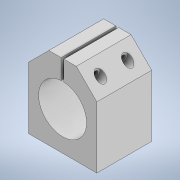
# Autodesk Inventor part: Motor_ParallelMecha_Fixation_Holder
Saved by Autodesk Inventor 2022 (Build 260153000, 153)
## iProperties
Created: 2022-07-26
Part Number: Motor_ParallelMecha_Fixation_Holder
Material: Generisch
Document SubType Name: Modeling
Designer: alexw
Density: 1 g/cm^3
Appearance: Vorgabe
Mass: 35.2121 g
Surface Area: 107.982 cm^2
Volume: 35.2121 cm^3
Hole_Dist2Center: 10,000 mm
Author: alexw
Autodesk Inventor part; units mm, degrees
note: some values were not read from the file. Chosen so that the rebuilt part matches the saved one: direction of "Bohrung2".
sketch "Skizze1" plane through (0, 0, 0) normal (0, 0, 1) x (1, 0, 0)
  line L0 (0, 0) -> (50, 0)
  line L1 (50, 0) -> (50, 45)
  line L2 (35, 60) -> (15, 60)
  line L3 (0, 45) -> (0, 0)
  circle A0 centre (25, 28) radius 17.5
  line L4 (25, 28) -> (25, 0) construction
  line L5 (0, 45) -> (15, 60)
  line L6 (35, 60) -> (50, 45)
  line L7 (24, 60) -> (26, 60)
  line L8 (26, 60) -> (26, 28)
  line L9 (26, 28) -> (24, 28)
  line L10 (24, 28) -> (24, 60)
  point P0 (50, 60)
  point P1 (0, 60)
  point P2 (25, 60)
  dimension "d0" = 50
  dimension "d1" = 35
  dimension "d2" = 60
  dimension "d3" = 15
  dimension "d4" = 15
  dimension "d5" = 15
  dimension "d6" = 15
  dimension "d7" = 28
  dimension "d10" = 2
  constraints: 22 end point, 4 midpoint, 4 parallel, 4 point on line, 2 horizontal, 2 perpendicular, 1 centre point, 1 vertical
  measures "d0" distance between parallel lines of L1 L3
  measures "d1" diameter of A0
  measures "d2" distance between parallel lines of L2 L0
  measures "d3" distance of L3.start point (0, 60)
  measures "d4" distance of L2.end point (0, 60)
  measures "d5" distance of L2.start point (50, 60)
  measures "d6" distance of L1.end point (50, 60)
  measures "d7" distance of L4.start L4.end
  measures "d10" distance between parallel lines of L8 L10
extrude "Extrusion1" add sketch "Skizze1" along normal blind 40 contours L3 L5 L2 L10 A0 L8 L6 L1 L0 | L2 L8 A0 L10
extrude "Extrusion2" cut sketch "Skizze1" along normal up to surface (40 mm away) contours L2 L8 A0 L10 | A0 L8 L9 L10 picked at (24.8888, 33.8323)
sketch "Skizze2" plane through (0, 0, 0) normal (0, -1, 0) x (1, 0, 0)
  line L0 (0, 0) -> (0, 40) construction
  line L1 (50, 0) -> (50, 40) construction
  line L2 (0, 40) -> (50, 40) construction
  line L3 (0, 0) -> (0, 40) construction
  line L4 (25, 20) -> (25, 40) construction
  line L5 (7.5, 40) -> (42.5, 40) construction
  line L6 (11, 20) -> (39, 20) construction
  point P0 (26, 40)
  point P1 (24, 40)
  point P2 (0, 20)
  dimension "d13" = 28
  constraints: 4 end point, 3 midpoint, 2 coincident, 1 horizontal, 1 point on line, 1 vertical
  measures "d13" distance of L6.start L6.end
hole "Bohrung1" at (11, 0, 20) at (39, 0, 20) direction (0, 1, 0) diameter 2.459 depth 10 tip angle 118 thread size "M3x0.5" class "6H" standard "ISO Metric profile"
ref_plane "Arbeitsebene1" through (42.5, 0, 0) normal (1, 0, 0) x (0, 0, -1)
sketch "Skizze3" plane through (42.5, 0, 0) normal (1, 0, 0) x (0, 0, -1)
  line L0 (0, 60) -> (-40, 60) construction
  line L1 (0, 45) -> (-40, 45) construction
  line L2 (-40, 45) -> (-40, 60) construction
  line L3 (-40, 52.5) -> (0, 52.5) construction
  line L4 (0, 45) -> (0, 60) construction
  point P0 (0, 0)
  point P1 (-20, 52.5)
  point P2 (-30, 52.5)
  point P3 (-10, 52.5)
  dimension "d44" = 10
  dimension "d45" = 10
  constraints: 3 midpoint, 2 end point, 2 point on line
  measures "d44" distance of point (-30, 52.5) point (-20, 52.5)
  measures "d45" distance of point (-20, 52.5) point (-10, 52.5)
ref_plane "Arbeitsebene2" through (0, 0, 20) normal (0, 0, 1) x (1, 0, 0)
ref_plane "Arbeitsebene3" through (0, 0, 30) normal (0, 0, 1) x (1, 0, 0)
ref_plane "Arbeitsebene4" through (0, 0, 10) normal (0, 0, -1) x (-1, 0, 0)
sketch "Skizze5" plane through (50, 0, 40) normal (1, 0, 0) x (0, 0, -1)
  line L0 (20, -12) -> (20, 72) construction
  line L1 (10, -12) -> (10, 72) construction
  line L2 (30, 72) -> (30, -12) construction
  point P0 (40, 0)
  dimension "Hole_Dist2Center" = 10
  dimension "d37" = 10
  measures "Hole_Dist2Center" distance between parallel lines of L0 L1
  measures "d37" distance between parallel lines of L2 L0
hole "Bohrung2" at (42.5, 52.5, 30) at (42.5, 52.5, 10) direction (-1, 0, 0) diameter 3.4 depth 18.5 counterbore diameter 6.5 counterbore depth 3.4 clearance for "Inbusschraube DIN EN ISO 4762" size "M3" standard "DIN"
delete faces "Fläche löschen1" heal yes whole lump no faces at (42.5, 50.5955, 29.1479) (42.5, 51.6084, 10.6154)
sketch "Skizze4" plane through (24, 45.4714, 0) normal (1, 0, 0) x (0, 0, -1)
  line L0 (-20, 7.0286) -> (-30, 7.0286) construction
  line L1 (-30, -57.4714) -> (-30, 26.5286) construction
  line L2 (-10, 26.5286) -> (-10, -57.4714) construction
  point P0 (0, -45.4714)
  point P1 (-10, 7.0286)
  constraints: 3 point on line, 2 end point, 1 coincident, 1 horizontal
hole "Bohrung3" at (24, 52.5, 30) at (24, 52.5, 10) direction (-1, 0, 0) diameter 3.242 end through all thread size "M4x0.7" class "6H" standard "ISO Metric profile"
equation "\"d0\" = Fixation_Width"
equation "\"d4\" = d3"
equation "\"d5\" = d3"
equation "\"d6\" = d5"
equation "\"d8\" = Fixation_Thickness"
equation "\"d11\" = Fixation_Thickness"
equation "\"d13\" = FixationHole_Dist"
equation "\"d44\" = Hole_Dist2Center"
equation "\"d45\" = d44"
equation "\"Fixation_Thickness\" = 40"
equation "\"Fixation_Width\" = 50"
equation "\"FixationHole_Dist\" = 28"
equation "\"d21\" = -0.5 * d5"
